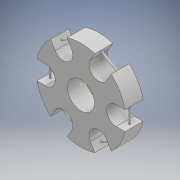
# Autodesk Inventor part: Holder
Saved by Autodesk Inventor 2018 (Build 220112000, 112)
## iProperties
Created: 2019-06-02
Part Number: Holder
Material: Generic
Document SubType Name: Modeling
Designer: dell
Density: 1 g/cm^3
Appearance: Default
Author: dell
Autodesk Inventor part; units mm, degrees
ref_plane "YZ Plane" through (0, 0, 0) normal (1, 0, 0) x (0, 1, 0)
ref_plane "XY Plane" through (0, 0, 0) normal (0, 0, 1) x (1, 0, 0)
sketch "Sketch1" plane through (0, 0, 0) normal (0, 1, 0) x (-1, 0, 0)
  circle A0 centre (0, 0) radius 50
  dimension "d0" = 100
  constraints: 1 centre point, 1 coincident
  measures "d0" diameter of A0
extrude "Extrusion1" add sketch "Sketch1" along normal blind 20
sketch "Sketch2" plane through (0, 20, 0) normal (0, 1, 0) x (1, 0, 0)
  line L0 (60.9024, 0) -> (39.0976, 0) construction
  circle A0 centre (0, 0) radius 50 projected
  line L1 (60.9024, 10.5) -> (39.0976, 10.5)
  line L2 (39.0976, -10.5) -> (60.9024, -10.5)
  arc A1 (60.9024, -10.5) -> (60.9024, 10.5) centre (60.9024, 0) ccw
  arc A2 (39.0976, 10.5) -> (39.0976, -10.5) centre (39.0976, 0) ccw
  point P0 (50, 0)
  dimension "d3" = 21
  constraints: 8 end point, 4 point on circle, 4 tangent, 2 centre point, 1 horizontal, 1 horizontal alignment, 1 midpoint, 1 parallel, 1 other
  measures "d3" diameter of A2
extrude "Extrusion2" cut sketch "Sketch2" against normal blind 20 contours A0 L2 A2 L1 | A0 L1 A1 L2 picked at (42.7317, 0)
pattern_circular "Circular Pattern1" count 6 over 360 about axis through (0, -10, 0) along (0, 1, 0) of "Extrusion2"
sketch "Sketch3" plane through (48.8851, 20, 10.5) normal (0, 0, -1) x (-1, 0, 0)
  point P0 (48.8851, -20)
sketch "Sketch4" plane through (0, 20, 0) normal (0, 1, 0) x (1, 0, 0)
  point P0 (0, 0)
ref_plane "Work Plane1" through (0, 10, 0) normal (0, 1, 0) x (-1, 0, 0)
sketch "Sketch5" plane through (0, 10, 0) normal (0, 1, 0) x (-1, 0, 0)
  line L0 (-15.3493, 47.5857) -> (-10.4555, 39.1095) projected
  arc A0 (-28.6421, 28.6095) -> (-10.4555, 39.1095) centre (-19.5488, 33.8595) ccw projected
  line L1 (-28.6421, 28.6095) -> (-33.5358, 37.0857) projected
  arc A1 (-33.5358, 37.0857) -> (-48.8851, 10.5) centre (0, 0) ccw projected
  line L2 (-48.8851, 10.5) -> (-39.0976, 10.5) projected
  arc A2 (-39.0976, -10.5) -> (-39.0976, 10.5) centre (-39.0976, 0) ccw projected
  line L3 (-39.0976, -10.5) -> (-48.8851, -10.5) projected
  arc A3 (-48.8851, -10.5) -> (-33.5358, -37.0857) centre (0, 0) ccw projected
  line L4 (-33.5358, -37.0857) -> (-28.6421, -28.6095) projected
  arc A4 (-10.4555, -39.1095) -> (-28.6421, -28.6095) centre (-19.5488, -33.8595) ccw projected
  line L5 (-10.4555, -39.1095) -> (-15.3493, -47.5857) projected
  arc A5 (-15.3493, -47.5857) -> (15.3493, -47.5857) centre (0, 0) ccw projected
  line L6 (15.3493, -47.5857) -> (10.4555, -39.1095) projected
  arc A6 (28.6421, -28.6095) -> (10.4555, -39.1095) centre (19.5488, -33.8595) ccw projected
  line L7 (28.6421, -28.6095) -> (33.5358, -37.0857) projected
  arc A7 (33.5358, -37.0857) -> (48.8851, -10.5) centre (0, 0) ccw projected
  line L8 (48.8851, -10.5) -> (39.0976, -10.5) projected
  arc A8 (39.0976, 10.5) -> (39.0976, -10.5) centre (39.0976, 0) ccw projected
  line L9 (39.0976, 10.5) -> (48.8851, 10.5) projected
  arc A9 (48.8851, 10.5) -> (33.5358, 37.0857) centre (0, 0) ccw projected
  line L10 (33.5358, 37.0857) -> (28.6421, 28.6095) projected
  arc A10 (10.4555, 39.1095) -> (28.6421, 28.6095) centre (19.5488, 33.8595) ccw projected
  line L11 (10.4555, 39.1095) -> (15.3493, 47.5857) projected
  arc A11 (15.3493, 47.5857) -> (-15.3493, 47.5857) centre (0, 0) ccw projected
  line L12 (15.3493, -47.5857) -> (10.4555, -39.1095) projected
  line L13 (12.9024, -43.3476) -> (31.0889, -32.8476)
  line L14 (28.6421, -28.6095) -> (33.5358, -37.0857) projected
  line L15 (43.9913, -10.5) -> (43.9913, 10.5)
  line L16 (31.0889, 32.8476) -> (12.9024, 43.3476)
  line L17 (15.3493, 47.5857) -> (10.4555, 39.1095) projected
  line L18 (-10.4555, 39.1095) -> (-15.3493, 47.5857) projected
  line L19 (-12.9024, 43.3476) -> (-31.0889, 32.8476)
  line L20 (-39.0976, 10.5) -> (-48.8851, 10.5) projected
  line L21 (-43.9913, 10.5) -> (-43.9913, -10.5)
  line L22 (-28.6421, -28.6095) -> (-33.5358, -37.0857) projected
  line L23 (-31.0889, -32.8476) -> (-12.9024, -43.3476)
  line L24 (-15.3493, -47.5857) -> (-10.4555, -39.1095) projected
  constraints: 12 end point, 12 midpoint
sketch "Sketch6" plane through (-15.3493, 0, 47.5857) normal (-0.866, 0, -0.5) x (-0.5, 0, 0.866)
  point P0 (-48.8851, 0)
sketch "Sketch7" plane through (15.3493, 0, 47.5857) normal (0.866, 0, -0.5) x (-0.5, 0, -0.866)
  line L0 (0, 10) -> (9.7874, 10) projected
  circle A0 centre (4.8937, 10) radius 1
  point P0 (48.8851, 0)
  dimension "d10" = 2
  constraints: 1 centre point, 1 coincident
  measures "d10" diameter of A0
sweep "Sweep1" add profiles "Sketch7" path "Sketch5" path curves L19
pattern_circular "Circular Pattern2" count 6 over 360 about axis through (0, -10, 0) along (0, 1, 0) of "Sweep1"
sketch "Sketch8" plane through (0, 0, 0) normal (0, -1, 0) x (1, 0, 0)
  circle A0 centre (0, 0) radius 15
  dimension "d16" = 30
  constraints: 1 centre point, 1 coincident
  measures "d16" diameter of A0
extrude "Extrusion3" cut sketch "Sketch8" against normal up to next
body "Solid1"
